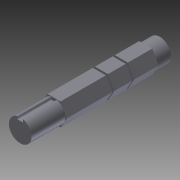
# Autodesk Inventor part: output_shaft
Saved by Autodesk Inventor 2012 (Build 160160000, 160)
## iProperties
Created: 2012-01-29
Part Number: output_shaft
Material: Steel
Document SubType Name: Modeling
Designer: Antonella Wilby
Mass: 83.5531 g
Surface Area: 36.3171 cm^2
Volume: 10.6437 cm^3
Density: 7.85 g/cm^3
Author: Antonella Wilby
Autodesk Inventor part; units mm, degrees
ref_plane "YZ Plane" through (0, 0, 0) normal (1, 0, 0) x (0, 1, 0)
sketch "Sketch1" plane through (0, 0, 0) normal (0, 0, 1) x (1, 0, 0)
  line L0 (-3.666174, 6.35) -> (3.666174, 6.35)
  line L1 (3.666174, 6.35) -> (7.332348, 0)
  line L2 (7.332348, 0) -> (3.666174, -6.35)
  line L3 (3.666174, -6.35) -> (-3.666174, -6.35)
  line L4 (-3.666174, -6.35) -> (-7.332348, 0)
  line L5 (-7.332348, 0) -> (-3.666174, 6.35)
  line L6 (-10.265288, 0) -> (10.265288, 0)
  line L7 (0, -8.89) -> (0, 8.89)
  point P0 (0, 0)
  point P1 (0, 0)
  dimension "d0" = 12.7
  constraints: 12 end point, 1 coincident, 1 perpendicular, 13 other
  measures "d0" distance between parallel lines of L0 L3
extrude "Extrusion1" add sketch "Sketch1" along normal mid plane 78.5622
sketch "Sketch5" plane through (0, 0, 39.2811) normal (0, 0, 1) x (1, 0, 0)
  line L0 (3.666174, 6.35) -> (7.332348, 0)
  line L1 (-3.666174, 6.35) -> (3.666174, 6.35)
  line L2 (-7.332348, 0) -> (-3.666174, 6.35)
  line L3 (-3.666174, -6.35) -> (-7.332348, 0)
  line L4 (3.666174, -6.35) -> (-3.666174, -6.35)
  line L5 (7.332348, 0) -> (3.666174, -6.35)
  circle A0 centre (0, 0) radius 6.35
  constraints: 1 centre point, 1 coincident, 1 tangent
extrude "Bearing Insert" cut sketch "Sketch5" against normal blind 7.9502 contours L0 A0 L1 | L0 L5 A0 | A0 L2 L1 | A0 L3 L2 | L5 L4 A0 | A0 L4 L3
mirror "Bearing Insert Mirror" about plane through (0, 0, 0) normal (0, 0, 1) of "Bearing Insert"
sketch "Sketch6" plane through (0, 0, -39.2811) normal (0, 0, -1) x (-1, 0, 0)
  circle A0 centre (0, 0) radius 6.35 projected
  circle A1 centre (0, 0) radius 3.175
  dimension "d11" = 6.35
  constraints: 1 centre point, 1 coincident
  measures "d11" diameter of A1
extrude "Extrusion5" cut sketch "Sketch6" against normal blind 15.875 contours A1
ref_plane "Work Plane2" through (3.666174, 6.35, -16.4719) normal (0, 0, -1) x (-1, 0, 0)
sketch "Sketch7" plane through (3.666174, 6.35, -16.4719) normal (0, 0, -1) x (-1, 0, 0)
  line L0 (0, 0) -> (3.666174, 0)
  line L1 (-1.833087, -3.175) -> (0, 0)
  circle A0 centre (3.666174, -6.35) radius 5.0292
  circle A1 centre (3.666174, -6.35) radius 7.332348
  dimension "d16" = 10.0584
  constraints: 2 coincident, 1 centre point, 3 other
  measures "d16" diameter of A0
extrude "Extrusion6" cut sketch "Sketch7" along normal blind 1.1684
ref_plane "Work Plane3" through (0, 0, -6.4389) normal (0, 0, -1) x (-1, 0, 0)
sketch "Sketch8" plane through (0, 0, -6.4389) normal (0, 0, -1) x (-1, 0, 0)
  line L0 (5.499261, 3.175) -> (7.332348, 0)
  line L1 (7.332348, 0) -> (5.499261, -3.175)
  circle A0 centre (0, 0) radius 5.0292
  circle A1 centre (0, 0) radius 7.332348
  point P0 (0, 0)
  dimension "d20" = 10.0584
  constraints: 2 coincident, 1 centre point, 1 horizontal alignment, 2 other
  measures "d20" diameter of A0
extrude "Extrusion7" cut sketch "Sketch8" against normal blind 1.1684
sketch "Sketch9" plane through (0, 0, 39.2811) normal (0, 0, 1) x (1, 0, 0)
  circle A0 centre (0, 0) radius 6.35
  line L0 (-3.666174, 6.35) -> (0, 6.35)
  line L1 (-5.499261, 3.175) -> (-3.666174, 6.35)
  circle A1 centre (0, 0) radius 7.332348
  constraints: 1 coincident, 3 other
sketch "Sketch9 outline for Extrusion8" plane through (0, 0, 39.2811) normal (0, 0, 1) x (1, 0, 0)
  circle A0 centre (0, 0) radius 7.332348
  arc A1 (-5.499261, 3.175) -> (0, 6.35) centre (0, 0) ccw
  arc A2 (0, 6.35) -> (-5.499261, 3.175) centre (0, 0) ccw
extrude "Extrusion8" cut sketch "Sketch9 outline for Extrusion8" against normal blind 19.05
sketch "Sketch10" plane through (0, 0, 39.2811) normal (0, 0, 1) x (1, 0, 0)
  circle A0 centre (0, 0) radius 6.35
  line L0 (-1.5875, 6.148361) -> (-1.5875, 4.560861)
  line L1 (-1.5875, 4.560861) -> (1.5875, 4.560861)
  line L2 (1.5875, 4.560861) -> (1.5875, 6.148361)
  line L3 (-10.265288, 0) -> (10.265288, 0)
  line L4 (0, -8.89) -> (0, 8.89)
  point P0 (0, 4.560861)
  dimension "d25" = 3.175
  dimension "d26" = 1.5875
  constraints: 6 end point, 2 perpendicular, 2 point on circle, 1 midpoint, 1 vertical, 1 vertical alignment
  measures "d25" distance of L0.end L1.end
  measures "d26" distance of L1.end L2.end
extrude "Extrusion9" cut sketch "Sketch10" against normal up to surface (19.05 mm away) contours L2 L1 L4 A0 | L4 L1 L0 A0
equation "\"d26\" = 0.5 * d25"
body "Solid1"
